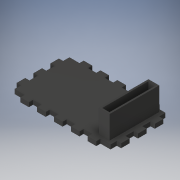
# Autodesk Inventor part: top
Saved by Autodesk Inventor 2019 (Build 230136000, 136)
## iProperties
Created: 2018-06-06
Part Number: top
Material: PBT Plastic Black
Document SubType Name: Modeling
Designer: stra92745
Density: 1.31 g/cm^3
Appearance: Smooth - White
Author: stra92745
Autodesk Inventor part; units mm, degrees
ref_plane "YZ Plane" through (0, 0, 0) normal (1, 0, 0) x (0, 1, 0)
ref_plane "XZ Plane" through (0, 0, 0) normal (0, 1, 0) x (-1, 0, 0)
ref_plane "XY Plane" through (0, 0, 0) normal (0, 0, 1) x (1, 0, 0)
sketch "Sketch1" plane through (0, 0, 0) normal (0, 1, 0) x (-1, 0, 0)
  line L0 (0, 0) -> (-99, 0)
  line L1 (-99, 0) -> (-99, -60)
  line L2 (-99, -60) -> (0, -60)
  line L3 (0, -60) -> (0, 0)
  line L4 (-83, -52) -> (-90, -52)
  line L5 (-90, -52) -> (-90, -8)
  line L6 (-90, -8) -> (-83, -8)
  line L7 (-83, -8) -> (-83, -52)
  dimension "d0" = 99
  dimension "d1" = 60
  dimension "d2" = 7
  dimension "d3" = 44
  dimension "d4" = 8
  dimension "d5" = 9
  constraints: 16 end point, 4 parallel, 2 horizontal, 2 perpendicular
  measures "d0" distance of L2.end L1.end
  measures "d1" distance of L1.end L0.end
  measures "d2" distance of L5.end L6.end
  measures "d3" distance of L6.end L4.start
  measures "d4" distance between parallel lines of L0 L6
  measures "d5" distance between parallel lines of L1 L5
extrude "Extrusion1" add sketch "Sketch1" along normal blind 4
sketch "Sketch2" plane through (0, 4, 0) normal (0, 1, 0) x (1, 0, 0)
  line L0 (83, 8) -> (83, 52) projected
  line L1 (83, 52) -> (90, 52) projected
  line L2 (90, 52) -> (90, 8) projected
  line L3 (90, 8) -> (83, 8) projected
  line L4 (91.5, 53.5) -> (81.5, 53.5)
  line L5 (81.5, 53.5) -> (81.5, 6.5)
  line L6 (81.5, 6.5) -> (91.5, 6.5)
  line L7 (91.5, 6.5) -> (91.5, 53.5)
  point P0 (0, 0)
  dimension "d8" = 1.5
  constraints: 8 end point, 3 other
  measures "d8" distance between parallel lines of L1 L4
extrude "Extrusion2" add sketch "Sketch2" along normal blind 22
sketch "Sketch3" plane through (0, 4, 0) normal (0, 1, 0) x (1, 0, 0)
  line L0 (99, 60) -> (0, 60) construction
  line L1 (0, 60) -> (0, 0) construction
  line L2 (0, 0) -> (99, 0) construction
  line L3 (99, 0) -> (99, 60) construction
  line L4 (4, 56) -> (95, 56) construction
  line L5 (95, 56) -> (95, 4) construction
  line L6 (95, 4) -> (4, 4) construction
  line L7 (4, 4) -> (4, 56) construction
  line L8 (0, 30) -> (99, 30) construction
  line L9 (49.5, 0) -> (49.5, 60) construction
  line L10 (0, 50) -> (0, 60)
  line L11 (0, 60) -> (13.5, 60)
  line L12 (13.5, 60) -> (13.5, 56)
  line L13 (13.5, 56) -> (4, 56)
  line L14 (4, 56) -> (4, 50)
  line L15 (4, 50) -> (0, 50)
  line L16 (0, 34) -> (4, 34)
  line L17 (4, 34) -> (4, 42)
  line L18 (4, 42) -> (0, 42)
  line L19 (0, 42) -> (0, 34)
  line L20 (45.5, 56) -> (37.5, 56)
  line L21 (37.5, 56) -> (37.5, 60)
  line L22 (37.5, 60) -> (45.5, 60)
  line L23 (45.5, 60) -> (45.5, 56)
  line L24 (29.5, 56) -> (21.5, 56)
  line L25 (21.5, 56) -> (21.5, 60)
  line L26 (21.5, 60) -> (29.5, 60)
  line L27 (29.5, 60) -> (29.5, 56)
  line L28 (0, 10) -> (0, 0)
  line L29 (0, 0) -> (13.5, 0)
  line L30 (13.5, 0) -> (13.5, 4)
  line L31 (13.5, 4) -> (4, 4)
  line L32 (4, 4) -> (4, 10)
  line L33 (4, 10) -> (0, 10)
  line L34 (0, 26) -> (4, 26)
  line L35 (4, 26) -> (4, 18)
  line L36 (4, 18) -> (0, 18)
  line L37 (0, 18) -> (0, 26)
  line L38 (45.5, 4) -> (37.5, 4)
  line L39 (37.5, 4) -> (37.5, 0)
  line L40 (37.5, 0) -> (45.5, 0)
  line L41 (45.5, 0) -> (45.5, 4)
  line L42 (29.5, 4) -> (21.5, 4)
  line L43 (21.5, 4) -> (21.5, 0)
  line L44 (21.5, 0) -> (29.5, 0)
  line L45 (29.5, 0) -> (29.5, 4)
  line L46 (99, 60) -> (99, 0) construction
  line L47 (95, 4) -> (95, 56) construction
  line L48 (99, 50) -> (99, 60)
  line L49 (99, 60) -> (85.5, 60)
  line L50 (85.5, 60) -> (85.5, 56)
  line L51 (85.5, 56) -> (95, 56)
  line L52 (95, 56) -> (95, 50)
  line L53 (95, 50) -> (99, 50)
  line L54 (99, 34) -> (95, 34)
  line L55 (95, 34) -> (95, 42)
  line L56 (95, 42) -> (99, 42)
  line L57 (99, 42) -> (99, 34)
  line L58 (53.5, 56) -> (61.5, 56)
  line L59 (61.5, 56) -> (61.5, 60)
  line L60 (61.5, 60) -> (53.5, 60)
  line L61 (53.5, 60) -> (53.5, 56)
  line L62 (69.5, 56) -> (77.5, 56)
  line L63 (77.5, 56) -> (77.5, 60)
  line L64 (77.5, 60) -> (69.5, 60)
  line L65 (69.5, 60) -> (69.5, 56)
  line L66 (77.5, 4) -> (77.5, 0)
  line L67 (69.5, 4) -> (77.5, 4)
  line L68 (77.5, 0) -> (69.5, 0)
  line L69 (69.5, 0) -> (69.5, 4)
  line L70 (61.5, 4) -> (61.5, 0)
  line L71 (53.5, 0) -> (53.5, 4)
  line L72 (53.5, 4) -> (61.5, 4)
  line L73 (61.5, 0) -> (53.5, 0)
  line L74 (85.5, 0) -> (85.5, 4)
  line L75 (85.5, 4) -> (95, 4)
  line L76 (95, 4) -> (95, 10)
  line L77 (99, 0) -> (85.5, 0)
  line L78 (99, 10) -> (99, 0)
  line L79 (95, 10) -> (99, 10)
  line L80 (95, 18) -> (99, 18)
  line L81 (95, 26) -> (95, 18)
  line L82 (99, 18) -> (99, 26)
  line L83 (99, 26) -> (95, 26)
  dimension "d11" = 4
  dimension "d12" = 8
  dimension "d13" = 4
  dimension "d14" = 8
  dimension "d15" = 8
  dimension "d16" = 4
  dimension "d17" = 8
  dimension "d18" = 8
  dimension "d19" = 8
  constraints: 160 end point, 48 symmetric about line, 14 point on line, 6 parallel, 5 perpendicular, 4 midpoint, 3 horizontal, 2 collinear, 3 other
  measures "d11" distance between parallel lines of L0 L4
  measures "d12" distance of L16.end L17.end
  measures "d13" distance between parallel lines of L8 L16
  measures "d14" distance between parallel lines of L15 L18
  measures "d15" distance of L20.start L20.end
  measures "d16" distance between parallel lines of L9 L23
  measures "d17" distance of L24.start L24.end
  measures "d18" distance between parallel lines of L21 L27
  measures "d19" distance between parallel lines of L12 L25
extrude "Extrusion3" cut sketch "Sketch3" against normal up to surface (4 mm away)
body "Solid1"
